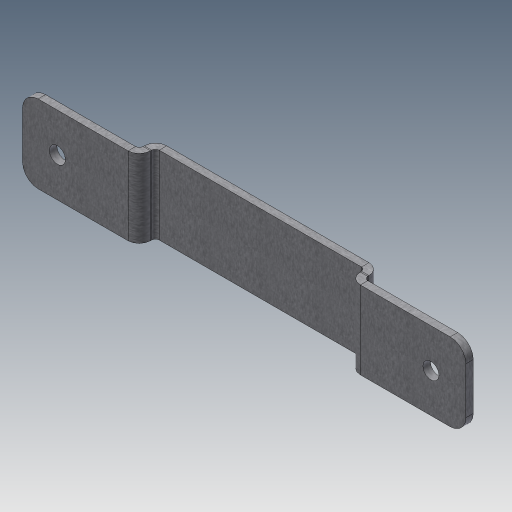
# Autodesk Inventor part: J010308
Saved by Autodesk Inventor 2023.4 (Build 274418000, 418)
## iProperties
RuleStatus: InUse
AfterDocSave0: file://Part Number Cleaner
Created: 2021-08-25
Material: STAINLESS STEEL, 316
Catalog Web Link: https://www.janelia.org/
Vendor: HHMI: JRC - JET
Document SubType Name: Sheet Metal
Designer: goulett
Density: 8 g/cm^3
Sheet Metal Rule: Default
Appearance: Metal-Steel (Stainless, Brushed)
Part Number: J010308
Project: COMMON
Description: CARD HOLDER BRACKET
DESIGN DEPARTMENT: HHMI: JRC - ID&F
SPECIAL FINISH: NONE
LAB/DEPT: COMMON
REQUESTING SCIENTIST: COMMON
SURFACE ROUGHNESS: 125Ra
Thickness: 0.060 in
ALTERED ITEM PART NUMBER: N/A
ALTERED ITEM VENDOR: N/A
ALTERED ITEM DESCRIPTION: N/A
PART NUMBER - LEGACY: Sheet Metal
Author: goulett
Revision Number: -
Autodesk Inventor part; units mm, degrees
note: some values were not read from the file. Chosen so that the rebuilt part matches the saved one: flange form of "Plate3".
ref_plane "YZ Plane" through (0, 0, 0) normal (1, 0, 0) x (0, 1, 0)
ref_plane "XZ Plane" through (0, 0, 0) normal (0, 1, 0) x (-1, 0, 0)
ref_plane "XY Plane" through (0, 0, 0) normal (0, 0, 1) x (1, 0, 0)
sketch "Sketch1" plane through (0, 0, 0) normal (0, 0, 1) x (1, 0, 0)
  line L0 (-20.6375, 7.9375) -> (20.6375, 7.9375)
  line L1 (20.6375, 7.9375) -> (20.6375, -7.9375)
  line L2 (20.6375, -7.9375) -> (-20.6375, -7.9375)
  line L3 (-20.6375, -7.9375) -> (-20.6375, 7.9375)
  point P0 (0, 0)
  point P1 (0, 7.9375)
  point P2 (-20.6375, 0)
  dimension "d0" = 41.275
  dimension "d1" = 15.875
  constraints: 8 end point, 2 midpoint, 2 parallel, 1 horizontal, 1 horizontal alignment, 1 perpendicular, 1 vertical alignment
  measures "d0" distance of L1.end L2.end
  measures "d1" distance of L0.end L1.end
extrude "Plate1" add sketch "Sketch1" along normal blind 1.524
sketch "Sketch3" plane through (-21.3995, -7.9375, 2.286) normal (-1, 0, 0) x (0, -1, 0)
  line L0 (-15.875, 0) -> (0, 0)
  line L1 (0, 0) -> (0, 0.254)
  line L2 (0, 0.254) -> (-15.875, 0.254)
  line L3 (-15.875, 0.254) -> (-15.875, 0)
  constraints: 6 end point, 1 horizontal, 1 perpendicular, 1 vertical
edge flange "Flange1" height 2.54 angle 90 thickness 1.524 bend radius 0.762 thickness toward (-1, 0, 0) relief tear relief width 1.524 relief depth 0.762 edges at (-20.6375, 0, 1.524) wall of the first edge with corners at (-21.3995, 7.9375, 2.286) (-21.3995, -7.9375, 2.286) (-21.3995, -7.9375, 2.54) (-21.3995, 7.9375, 2.54)
bend "Bend1"
corner "Corner1"
sketch "Sketch4" plane through (21.3995, 7.9375, 2.286) normal (1, 0, 0) x (0, 1, 0)
  line L0 (-15.875, 0) -> (0, 0)
  line L1 (0, 0) -> (0, 0.254)
  line L2 (0, 0.254) -> (-15.875, 0.254)
  line L3 (-15.875, 0.254) -> (-15.875, 0)
  constraints: 6 end point, 1 horizontal, 1 perpendicular, 1 vertical
edge flange "Flange2" height 2.54 angle 90 thickness 1.524 bend radius 0.762 thickness toward (1, 0, 0) relief tear relief width 1.524 relief depth 0.762 edges at (20.6375, 0, 1.524) wall of the first edge with corners at (21.3995, -7.9375, 2.286) (21.3995, 7.9375, 2.286) (21.3995, 7.9375, 2.54) (21.3995, -7.9375, 2.54)
bend "Bend2"
corner "Corner2"
sketch "Sketch7" plane through (-23.6855, 7.9375, 3.302) normal (0, 0, 1) x (1, 0, 0)
  line L0 (0, -15.875) -> (0, 0)
  line L1 (0, 0) -> (-21.5265, 0)
  line L2 (-21.5265, 0) -> (-21.5265, -15.875)
  line L3 (-21.5265, -15.875) -> (0, -15.875)
  constraints: 6 end point, 1 horizontal, 1 perpendicular, 1 vertical
edge flange "Flange5" height 23.8125 angle 90 thickness 1.524 bend radius 0.762 thickness toward (0, 0, 1) relief tear relief width 1.524 relief depth 0.762 edges at (-22.9235, 0, 2.54) wall of the first edge with corners at (-23.6855, -7.9375, 3.302) (-23.6855, 7.9375, 3.302) (-45.212, 7.9375, 3.302) (-45.212, -7.9375, 3.302)
bend "Bend5"
corner "Corner5"
sketch "Sketch8" plane through (23.6855, -7.9375, 3.302) normal (0, 0, 1) x (1, 0, 0)
  line L0 (0, 15.875) -> (0, 0)
  line L1 (0, 0) -> (21.5265, 0)
  line L2 (21.5265, 0) -> (21.5265, 15.875)
  line L3 (21.5265, 15.875) -> (0, 15.875)
  constraints: 6 end point, 1 horizontal, 1 perpendicular, 1 vertical
edge flange "Flange6" height 23.8125 angle 90 thickness 1.524 bend radius 0.762 thickness toward (0, 0, 1) relief tear relief width 1.524 relief depth 0.762 edges at (21.3995, 0, 2.54) wall of the first edge with corners at (23.6855, 7.9375, 3.302) (23.6855, -7.9375, 3.302) (45.212, -7.9375, 3.302) (45.212, 7.9375, 3.302)
bend "Bend6"
corner "Corner6"
sketch "Sketch9" plane through (-45.212, -7.9375, 3.302) normal (0, 0, -1) x (-1, 0, 0)
  line L0 (0, 0) -> (0, 15.875) projected
  point P0 (-45.212, 7.9375)
  point P1 (-7.112, 7.9375)
  point P2 (-83.312, 7.9375)
  point P3 (0, 7.9375)
  dimension "d65" = 76.2
  dimension "d66" = 7.112
  constraints: 2 horizontal alignment, 1 midpoint
  measures "d65" distance of point (-83.312, 7.938) point (-7.112, 7.938)
  measures "d66" distance from line of L0 point (-7.112, 7.938)
hole "Hole1" at (-38.1, 0, 3.302) at (38.1, 0, 3.302) direction (0, 0, 1) diameter 3.302 depth 1.524 tip angle 118
fillet "Corner Round1" radius 3.175 4 edges at (-45.212, -7.9375, 4.064) (-45.212, 7.9375, 4.064) (45.212, 7.9375, 4.064) (45.212, -7.9375, 4.064)
equation "\"d72\" = Thickness"
equation "\"d2\" = Thickness"
equation "\"d5\" = BendReliefWidth"
equation "\"d6\" = BendReliefDepth"
equation "\"d7\" = MinimumRemnant"
equation "\"d8\" = TransitionRadius"
equation "\"d12\" = CornerReliefSize"
equation "\"d13\" = GapSize"
equation "\"d14\" = JacobiRadiusSize"
equation "\"d15\" = BendReliefWidth"
equation "\"d16\" = BendReliefDepth"
equation "\"d17\" = MinimumRemnant"
equation "\"d18\" = TransitionRadius"
equation "\"d22\" = CornerReliefSize"
equation "\"d23\" = GapSize"
equation "\"d24\" = JacobiRadiusSize"
equation "\"d45\" = BendReliefWidth"
equation "\"d46\" = BendReliefDepth"
equation "\"d47\" = MinimumRemnant"
equation "\"d48\" = TransitionRadius"
equation "\"d52\" = CornerReliefSize"
equation "\"d53\" = GapSize"
equation "\"d54\" = JacobiRadiusSize"
equation "\"d55\" = BendReliefWidth"
equation "\"d56\" = BendReliefDepth"
equation "\"d57\" = MinimumRemnant"
equation "\"d58\" = TransitionRadius"
equation "\"d62\" = CornerReliefSize"
equation "\"d63\" = GapSize"
equation "\"d64\" = JacobiRadiusSize"
equation "\"BendRadius\" = Thickness"
equation "\"BendReliefWidth\" = Thickness"
equation "\"BendReliefDepth\" = 0.5 * Thickness"
equation "\"CornerReliefSize\" = 4 * Thickness"
equation "\"MinimumRemnant\" = 2 * Thickness"
equation "\"TransitionRadius\" = BendRadius"
equation "\"JacobiRadiusSize\" = BendRadius"
equation "\"GapSize\" = Thickness"
equation "\"Thickness\" = 1.524"
body "Solid1"
